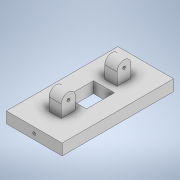
# Autodesk Inventor part: basePlate
Saved by Autodesk Inventor 2021 (Build 250183000, 183)
## iProperties
Created: 2022-09-16
Part Number: basePlate
Material: Generic
Document SubType Name: Modeling
Designer: ereg140
Density: 1 g/cm^3
Appearance: Default
Author: ereg140
Autodesk Inventor part; units mm, degrees
ref_plane "YZ Plane" through (0, 0, 0) normal (1, 0, 0) x (0, 1, 0)
ref_plane "XZ Plane" through (0, 0, 0) normal (0, 1, 0) x (-1, 0, 0)
ref_plane "XY Plane" through (0, 0, 0) normal (0, 0, 1) x (1, 0, 0)
sketch "Sketch1" plane through (0, 0, 0) normal (0, 1, 0) x (-1, 0, 0)
  line L0 (0, 0) -> (40, 0)
  line L1 (40, 0) -> (40, -80)
  line L2 (40, -80) -> (0, -80)
  line L3 (0, -80) -> (0, 0)
  dimension "d0" = 40
  dimension "d1" = 80
  constraints: 8 end point, 2 parallel, 1 horizontal, 1 perpendicular
  measures "d0" distance of L0.start L0.end
  measures "d1" distance of L2.end L0.start
extrude "Extrusion1" add sketch "Sketch1" along normal blind 8
sketch "Sketch2" plane through (0, 8, 0) normal (0, 1, 0) x (1, 0, 0)
  line L0 (-24.4, 15) -> (-15.6, 15)
  line L1 (-15.6, 15) -> (-15.6, 25)
  line L2 (-15.6, 25) -> (-24.4, 25)
  line L3 (-24.4, 25) -> (-24.4, 15)
  line L4 (-40, 0) -> (0, 0) projected
  line L5 (-24.4, 55) -> (-15.6, 55)
  line L6 (-15.6, 55) -> (-15.6, 65)
  line L7 (-15.6, 65) -> (-24.4, 65)
  line L8 (-24.4, 65) -> (-24.4, 55)
  line L9 (-20, 25) -> (-20, 55) construction
  line L10 (-40, 80) -> (-40, 0) construction
  point P0 (-20, 15)
  point P1 (-20, 0)
  point P2 (-20, 40)
  point P3 (-40, 40)
  dimension "d4" = 8.8
  dimension "d5" = 10
  dimension "d6" = 10
  dimension "d7" = 8.8
  dimension "d8" = 30
  constraints: 18 end point, 6 midpoint, 4 parallel, 2 horizontal, 2 perpendicular, 1 horizontal alignment, 1 vertical alignment
  measures "d4" distance between parallel lines of L1 L3
  measures "d5" distance between parallel lines of L2 L0
  measures "d6" distance between parallel lines of L7 L5
  measures "d7" distance between parallel lines of L6 L8
  measures "d8" distance between parallel lines of L5 L2
extrude "Extrusion2" add sketch "Sketch2" along normal blind 14
fillet "Fillet1" radius 5 4 edges at (-20, 22, -15) (-20, 22, -25) (-20, 22, -55) (-20, 22, -65)
sketch "Sketch3" plane through (-15.6, 8, -15) normal (1, 0, 0) x (0, 0, -1)
  arc A0 (10, 9) -> (0, 9) centre (5, 9) ccw projected
  circle A1 centre (5, 9) radius 1
  arc A2 (50, 9) -> (40, 9) centre (45, 9) ccw projected
  circle A3 centre (45, 9) radius 1
  point P0 (-15, -8)
  dimension "d12" = 2
  dimension "d13" = 2
  constraints: 2 centre point, 2 coincident
  measures "d12" diameter of A1
  measures "d13" diameter of A3
extrude "Extrusion3" cut sketch "Sketch3" against normal blind 14
sketch "Sketch4" plane through (-40, 0, 0) normal (0, 0, 1) x (1, 0, 0)
  circle A0 centre (20, 4) radius 1
  line L0 (40, 0) -> (40, 8) projected
  line L1 (0, 8) -> (40, 8) projected
  point P0 (40, 4)
  point P1 (20, 8)
  dimension "d16" = 2
  constraints: 2 midpoint, 1 centre point, 1 horizontal alignment, 1 vertical alignment
  measures "d16" diameter of A0
extrude "Extrusion4" cut sketch "Sketch4" against normal blind 5
sketch "Sketch5" plane through (0, 0, -80) normal (0, 0, -1) x (-1, 0, 0)
  circle A0 centre (20, 4) radius 1 projected
  point P0 (0, 0)
extrude "Extrusion5" cut sketch "Sketch5" against normal blind 5
sketch "Sketch6" plane through (0, 8, 0) normal (0, 1, 0) x (1, 0, 0)
  line L0 (-27.5, 50) -> (-12.5, 50)
  line L1 (-12.5, 50) -> (-12.5, 30)
  line L2 (-12.5, 30) -> (-27.5, 30)
  line L3 (-27.5, 30) -> (-27.5, 50)
  line L4 (-40, 80) -> (-40, 0) projected
  line L5 (-40, 0) -> (0, 0) projected
  point P0 (-12.5, 40)
  point P1 (-40, 40)
  point P2 (-20, 50)
  point P3 (-20, 0)
  dimension "d21" = 20
  dimension "d22" = 15
  constraints: 8 end point, 4 midpoint, 2 parallel, 1 horizontal, 1 horizontal alignment, 1 perpendicular, 1 vertical alignment
  measures "d21" distance of L0.end L1.end
  measures "d22" distance of L0.start L0.end
extrude "Extrusion6" cut sketch "Sketch6" against normal up to surface (8 mm away)
body "Solid1"
